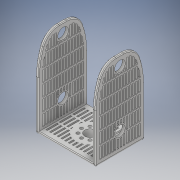
# Autodesk Inventor part: Wheel Case V2
Saved by Autodesk Inventor 2019 (Build 230136000, 136)
## iProperties
Created: 2018-12-01
Part Number: Wheel Case V2
Material: Generic
Document SubType Name: Modeling
Designer: Ashley
Density: 1 g/cm^3
Appearance: Default
Author: Ashley
Autodesk Inventor part; units mm, degrees
ref_plane "YZ Plane" through (0, 0, 0) normal (1, 0, 0) x (0, 1, 0)
ref_plane "XZ Plane" through (0, 0, 0) normal (0, 1, 0) x (-1, 0, 0)
ref_plane "XY Plane" through (0, 0, 0) normal (0, 0, 1) x (1, 0, 0)
sketch "Sketch1" plane through (0, 0, 0) normal (0, 1, 0) x (-1, 0, 0)
  line L0 (40, 32.5) -> (-40, 32.5)
  line L1 (-40, 32.5) -> (-40, -32.5)
  line L2 (-40, -32.5) -> (40, -32.5)
  line L3 (40, -32.5) -> (40, 32.5)
  line L4 (40, 32.5) -> (-40, -32.5) construction
  line L5 (-40, 32.5) -> (40, -32.5) construction
  point P0 (0, 0)
  dimension "d0" = 80
  dimension "d1" = 65
  constraints: 12 end point, 2 midpoint, 2 parallel, 1 horizontal, 1 perpendicular
  measures "d0" distance of L1.end L2.end
  measures "d1" distance of L0.end L1.end
extrude "Top Base Extrusion" add sketch "Sketch1" along normal blind 4
sketch "Sketch2" plane through (0, 4, 0) normal (0, 1, 0) x (1, 0, 0)
  line L0 (-40, -32.5) -> (40, -32.5) construction
  line L1 (40, -32.5) -> (40, 32.5) construction
  line L2 (-40, 32.5) -> (-40, -32.5) construction
  line L3 (-40, 32.5) -> (-36, 32.5)
  line L4 (-36, 32.5) -> (-36, -32.5)
  line L5 (-36, -32.5) -> (-40, -32.5)
  line L6 (-40, -32.5) -> (-40, 32.5)
  line L7 (40, 32.5) -> (36, 32.5)
  line L8 (36, 32.5) -> (36, -32.5)
  line L9 (36, -32.5) -> (40, -32.5)
  line L10 (40, -32.5) -> (40, 32.5)
  point P0 (0, 0)
  dimension "d4" = 4
  dimension "d5" = 4
  constraints: 16 end point, 4 parallel, 2 horizontal, 2 perpendicular, 2 point on line
  measures "d4" distance between parallel lines of L4 L2
  measures "d5" distance between parallel lines of L1 L8
extrude "Side Extrusions" add sketch "Sketch2" along normal blind 110
sketch "Sketch3" plane through (40, 0, 32.5) normal (1, 0, 0) x (0, 0, -1)
  circle A0 centre (32.5, 101.5) radius 7.1
  circle A1 centre (32.5, 26.5) radius 7
  line L0 (65, 0) -> (65, 114) construction
  line L1 (0, 114) -> (65, 114) construction
  line L2 (0, 0) -> (0, 114) construction
  line L3 (0, 4) -> (65, 4) construction
  point P0 (32.5, 0)
  dimension "d8" = 14.2
  dimension "d11" = 101.5
  dimension "d43" = 75
  dimension "d44" = 14
  dimension "d45" = 65
  dimension "d46" = 32.5
  dimension "d47" = 32.5
  dimension "d48" = 32.5
  dimension "d49" = 12.5
  dimension "d50" = 22.5
  constraints: 2 centre point
  measures "d8" diameter of A0
  measures "d11" distance of point (32.5, 0) A0.centre
  measures "d43" distance of A1.centre A0.centre
  measures "d44" diameter of A1
  measures "d45" distance between parallel lines of L2 L0
  measures "d46" distance from line of L0 A0.centre
  measures "d47" distance from line of L2 A0.centre
  measures "d48" distance from line of L0 A1.centre
  measures "d49" distance from line of A0.centre L1
  measures "d50" distance from line of A1.centre L3
extrude "Wheel Axel Hole" cut sketch "Sketch3" against normal up to surface (80 mm away)
sketch "Sketch4" plane through (0, 0, 0) normal (0, -1, 0) x (1, 0, 0)
  circle A0 centre (0, 0) radius 7.1
  circle A1 centre (0, 0) radius 16
  dimension "d16" = 14.2
  dimension "d17" = 32
  constraints: 2 centre point, 2 coincident
  measures "d16" diameter of A0
  measures "d17" diameter of A1
extrude "Chain Interferance Extrusion" add sketch "Sketch4" along normal blind 6
sketch "Sketch5" plane through (0, 0, 0) normal (0, -1, 0) x (1, 0, 0)
  circle A0 centre (0, 0) radius 7.1 construction
  circle A1 centre (0, 0) radius 7.1
  constraints: 1 centre point, 1 coincident, 1 concentric
extrude "Top Center Bearing Hole" cut sketch "Sketch5" against normal up to surface (4 mm away)
sketch "Sketch7" plane through (0, -6, 0) normal (0, -1, 0) x (1, 0, 0)
  circle A0 centre (0, 0) radius 7.1 construction
  circle A1 centre (0, 11.314) radius 2.05
  circle A2 centre (-8.0002, 8.0002) radius 2.05
  circle A3 centre (-11.314, 0) radius 2.05
  circle A4 centre (-8.0002, -8.0002) radius 2.05
  circle A5 centre (0, -11.314) radius 2.05
  circle A6 centre (8.0002, -8.0002) radius 2.05
  circle A7 centre (11.314, 0) radius 2.05
  circle A8 centre (8.0002, 8.0002) radius 2.05
  dimension "d23" = 4.1
  dimension "d24" = 11.314
  dimension "d27" = 360
  constraints: 8 centre point, 17 other
  measures "d23" diameter of A1
  measures "d24" distance of A0.centre A1.centre
extrude "Sprocket Screws Holes" cut sketch "Sketch7" against normal up to next
sketch "Sketch8" plane through (40, 0, 32.5) normal (1, 0, 0) x (0, 0, -1)
  line L0 (65, 0) -> (65, 114) construction
  line L1 (0, 114) -> (65, 114) construction
  line L2 (0, 0) -> (0, 114) construction
  line L3 (65, 91.5) -> (52.0096, 114)
  line L4 (65, 114) -> (0, 114) construction
  line L5 (65, 91.5) -> (90.9808, 91.5) construction
  line L6 (0, 91.5) -> (34.6363, 91.5) construction
  line L7 (0, 91.5) -> (44.4453, 91.5) construction
  line L8 (0, 91.5) -> (12.9904, 114)
  line L9 (65, 91.5) -> (65, 114)
  line L10 (52.0096, 114) -> (65, 114)
  line L11 (12.9904, 114) -> (0, 114)
  line L12 (0, 91.5) -> (0, 114)
  line L13 (0, 91.5) -> (-31.251, 91.5) construction
  point P0 (32.5, 0)
  dimension "d32" = 120
  dimension "d51" = 120
  constraints: 20 end point, 5 point on line, 3 collinear, 3 horizontal, 1 equal length, 1 perpendicular
  measures "d32" angle of L5 L3
  measures "d51" angle of L13 L8
extrude "Side Corners Cut" cut sketch "Sketch8" against normal up to surface (80 mm away)
fillet "Fillet1" radius 95 4 edges at (38, 91.5, 32.5) (-38, 91.5, 32.5) (38, 91.5, -32.5) (-38, 91.5, -32.5)
fillet "Fillet2" radius 23 4 edges at (38, 114, 19.5096) (38, 114, -19.5096) (-38, 114, -19.5096) (-38, 114, 19.5096)
fillet "Fillet3" radius 3 4 edges at (0, 0, -32.5) (-40, 0, 0) (40, 0, 0) (0, 0, 32.5)
fillet "Fillet4" radius 3 1 edges at (-16, 0, 0)
fillet "Fillet5" radius 1 1 edges at (-16, -6, 0)
fillet "Fillet7" radius 1 34 edges at (40, 109.8726, 18.1832) (40, 114, 0) (40, 109.8726, -18.1832) (40, 82.7695, -31.0162) (40, 34.5224, -32.5) (39.1213, 0.8787, -31.6213) (40, 34.5224, 32.5) (39.1213, 0.8787, 31.6213) (40, 82.7695, 31.0162) (36, 35.0224, 32.5) (36, 109.8726, 18.1832) (36, 114, 0) (36, 109.8726, -18.1832) (36, 82.7695, -31.0162) (36, 35.0224, -32.5) (36, 82.7695, 31.0162) (-36, 109.8726, 18.1832) (-36, 114, 0) (-36, 109.8726, -18.1832) (-36, 82.7695, -31.0162) (-36, 35.0224, -32.5) (-36, 35.0224, 32.5) (-36, 82.7695, 31.0162) (-40, 34.5224, 32.5) (-39.1213, 0.8787, 31.6213) (-40, 109.8726, 18.1832) (-40, 114, 0) (-40, 109.8726, -18.1832) (-40, 82.7695, -31.0162) (-40, 34.5224, -32.5) (-39.1213, 0.8787, -31.6213) (-40, 82.7695, 31.0162) (0, 4, 32.5) (0, 4, -32.5)
sketch "Sketch9" plane through (40, 3, -31.5) normal (1, 0, 0) x (0, 0, -1)
  circle A0 centre (-31.5, 98.5) radius 7.1 construction
  circle A1 centre (-31.5, 23.5) radius 7 construction
  line L0 (0, 63.0448) -> (0, 0) construction
  arc A2 (0, 63.0448) -> (-5.8268, 95.6252) centre (-94, 63.0448) ccw construction
  arc A3 (-5.8268, 95.6252) -> (-26.4631, 110) centre (-26.4631, 88) ccw construction
  line L1 (-36.5369, 110) -> (-26.4631, 110) construction
  arc A4 (-36.5369, 110) -> (-57.1732, 95.6252) centre (-36.5369, 88) ccw construction
  arc A5 (-57.1732, 95.6252) -> (-63, 63.0448) centre (31, 63.0448) ccw construction
  line L2 (-63, 0) -> (-63, 63.0448) construction
  line L3 (0, 0) -> (-63, 0) construction
  line L4 (-58.5, 4) -> (-56.5, 4)
  line L5 (-56.5, 4) -> (-56.5, 19)
  line L6 (-56.5, 19) -> (-58.5, 19)
  line L7 (-58.5, 19) -> (-58.5, 4)
  line L8 (-61, -3) -> (-2, -3) construction
  line L9 (-56.5, 36) -> (-58.5, 36)
  line L10 (-58.5, 21) -> (-56.5, 21)
  line L11 (-58.5, 36) -> (-58.5, 21)
  line L12 (-56.5, 21) -> (-56.5, 36)
  line L13 (-56.5, 53) -> (-58.5, 53)
  line L14 (-58.5, 38) -> (-56.5, 38)
  line L15 (-58.5, 53) -> (-58.5, 38)
  line L16 (-56.5, 38) -> (-56.5, 53)
  line L17 (-56.5, 70) -> (-58.5, 70)
  line L18 (-58.5, 55) -> (-56.5, 55)
  line L19 (-58.5, 70) -> (-58.5, 55)
  line L20 (-56.5, 55) -> (-56.5, 70)
  line L21 (-52.5, 19) -> (-54.5, 19)
  line L22 (-54.5, 4) -> (-52.5, 4)
  line L23 (-54.5, 19) -> (-54.5, 4)
  line L24 (-52.5, 4) -> (-52.5, 19)
  line L25 (-52.5, 36) -> (-54.5, 36)
  line L26 (-54.5, 21) -> (-52.5, 21)
  line L27 (-54.5, 36) -> (-54.5, 21)
  line L28 (-52.5, 21) -> (-52.5, 36)
  line L29 (-52.5, 53) -> (-54.5, 53)
  line L30 (-54.5, 38) -> (-52.5, 38)
  line L31 (-54.5, 53) -> (-54.5, 38)
  line L32 (-52.5, 38) -> (-52.5, 53)
  line L33 (-52.5, 70) -> (-54.5, 70)
  line L34 (-54.5, 55) -> (-52.5, 55)
  line L35 (-54.5, 70) -> (-54.5, 55)
  line L36 (-52.5, 55) -> (-52.5, 70)
  line L37 (-48.5, 19) -> (-50.5, 19)
  line L38 (-50.5, 4) -> (-48.5, 4)
  line L39 (-50.5, 19) -> (-50.5, 4)
  line L40 (-48.5, 4) -> (-48.5, 19)
  line L41 (-48.5, 36) -> (-50.5, 36)
  line L42 (-50.5, 21) -> (-48.5, 21)
  line L43 (-50.5, 36) -> (-50.5, 21)
  line L44 (-48.5, 21) -> (-48.5, 36)
  line L45 (-48.5, 53) -> (-50.5, 53)
  line L46 (-50.5, 38) -> (-48.5, 38)
  line L47 (-50.5, 53) -> (-50.5, 38)
  line L48 (-48.5, 38) -> (-48.5, 53)
  line L49 (-48.5, 70) -> (-50.5, 70)
  line L50 (-50.5, 55) -> (-48.5, 55)
  line L51 (-50.5, 70) -> (-50.5, 55)
  line L52 (-48.5, 55) -> (-48.5, 70)
  line L53 (-44.5, 19) -> (-46.5, 19)
  line L54 (-46.5, 4) -> (-44.5, 4)
  line L55 (-46.5, 19) -> (-46.5, 4)
  line L56 (-44.5, 4) -> (-44.5, 19)
  line L57 (-44.5, 36) -> (-46.5, 36)
  line L58 (-46.5, 21) -> (-44.5, 21)
  line L59 (-46.5, 36) -> (-46.5, 21)
  line L60 (-44.5, 21) -> (-44.5, 36)
  line L61 (-44.5, 53) -> (-46.5, 53)
  line L62 (-46.5, 38) -> (-44.5, 38)
  line L63 (-46.5, 53) -> (-46.5, 38)
  line L64 (-44.5, 38) -> (-44.5, 53)
  line L65 (-44.5, 70) -> (-46.5, 70)
  line L66 (-46.5, 55) -> (-44.5, 55)
  line L67 (-46.5, 70) -> (-46.5, 55)
  line L68 (-44.5, 55) -> (-44.5, 70)
  line L69 (-40.5, 19) -> (-42.5, 19)
  line L70 (-42.5, 4) -> (-40.5, 4)
  line L71 (-42.5, 19) -> (-42.5, 4)
  line L72 (-40.5, 4) -> (-40.5, 19)
  line L73 (-40.5, 36) -> (-42.5, 36)
  line L74 (-42.5, 21) -> (-40.5, 21)
  line L75 (-42.5, 36) -> (-42.5, 21)
  line L76 (-40.5, 21) -> (-40.5, 36)
  line L77 (-40.5, 53) -> (-42.5, 53)
  line L78 (-42.5, 38) -> (-40.5, 38)
  line L79 (-42.5, 53) -> (-42.5, 38)
  line L80 (-40.5, 38) -> (-40.5, 53)
  line L81 (-40.5, 70) -> (-42.5, 70)
  line L82 (-42.5, 55) -> (-40.5, 55)
  line L83 (-42.5, 70) -> (-42.5, 55)
  line L84 (-40.5, 55) -> (-40.5, 70)
  line L85 (-52.5, 87) -> (-54.5, 87)
  line L86 (-52.5, 72) -> (-52.5, 87)
  line L87 (-54.5, 87) -> (-54.5, 72)
  line L88 (-54.5, 72) -> (-52.5, 72)
  line L89 (-36.5, 55) -> (-36.5, 70)
  line L90 (-38.5, 70) -> (-38.5, 55)
  line L91 (-38.5, 55) -> (-36.5, 55)
  line L92 (-36.5, 70) -> (-38.5, 70)
  line L93 (-32.5, 55) -> (-32.5, 70)
  line L94 (-34.5, 55) -> (-32.5, 55)
  line L95 (-34.5, 70) -> (-34.5, 55)
  line L96 (-32.5, 70) -> (-34.5, 70)
  line L97 (-28.5, 55) -> (-28.5, 70)
  line L98 (-30.5, 55) -> (-28.5, 55)
  line L99 (-30.5, 70) -> (-30.5, 55)
  line L100 (-28.5, 70) -> (-30.5, 70)
  line L101 (-24.5, 55) -> (-24.5, 70)
  line L102 (-26.5, 55) -> (-24.5, 55)
  line L103 (-26.5, 70) -> (-26.5, 55)
  line L104 (-24.5, 70) -> (-26.5, 70)
  line L105 (-20.5, 55) -> (-20.5, 70)
  line L106 (-22.5, 55) -> (-20.5, 55)
  line L107 (-22.5, 70) -> (-22.5, 55)
  line L108 (-20.5, 70) -> (-22.5, 70)
  line L109 (-16.5, 55) -> (-16.5, 70)
  line L110 (-18.5, 55) -> (-16.5, 55)
  line L111 (-18.5, 70) -> (-18.5, 55)
  line L112 (-16.5, 70) -> (-18.5, 70)
  line L113 (-12.5, 55) -> (-12.5, 70)
  line L114 (-14.5, 55) -> (-12.5, 55)
  line L115 (-14.5, 70) -> (-14.5, 55)
  line L116 (-12.5, 70) -> (-14.5, 70)
  line L117 (-8.5, 55) -> (-8.5, 70)
  line L118 (-10.5, 55) -> (-8.5, 55)
  line L119 (-10.5, 70) -> (-10.5, 55)
  line L120 (-8.5, 70) -> (-10.5, 70)
  line L121 (-4.5, 55) -> (-4.5, 70)
  line L122 (-6.5, 55) -> (-4.5, 55)
  line L123 (-6.5, 70) -> (-6.5, 55)
  line L124 (-4.5, 70) -> (-6.5, 70)
  line L125 (-36.5, 38) -> (-36.5, 53)
  line L126 (-38.5, 38) -> (-36.5, 38)
  line L127 (-38.5, 53) -> (-38.5, 38)
  line L128 (-36.5, 53) -> (-38.5, 53)
  line L129 (-32.5, 38) -> (-32.5, 53)
  line L130 (-34.5, 38) -> (-32.5, 38)
  line L131 (-34.5, 53) -> (-34.5, 38)
  line L132 (-32.5, 53) -> (-34.5, 53)
  line L133 (-28.5, 38) -> (-28.5, 53)
  line L134 (-30.5, 38) -> (-28.5, 38)
  line L135 (-30.5, 53) -> (-30.5, 38)
  line L136 (-28.5, 53) -> (-30.5, 53)
  line L137 (-24.5, 38) -> (-24.5, 53)
  line L138 (-26.5, 38) -> (-24.5, 38)
  line L139 (-26.5, 53) -> (-26.5, 38)
  line L140 (-24.5, 53) -> (-26.5, 53)
  line L141 (-20.5, 38) -> (-20.5, 53)
  line L142 (-22.5, 38) -> (-20.5, 38)
  line L143 (-22.5, 53) -> (-22.5, 38)
  line L144 (-20.5, 53) -> (-22.5, 53)
  line L145 (-16.5, 38) -> (-16.5, 53)
  line L146 (-18.5, 38) -> (-16.5, 38)
  line L147 (-18.5, 53) -> (-18.5, 38)
  line L148 (-16.5, 53) -> (-18.5, 53)
  line L149 (-12.5, 38) -> (-12.5, 53)
  line L150 (-14.5, 38) -> (-12.5, 38)
  line L151 (-14.5, 53) -> (-14.5, 38)
  line L152 (-12.5, 53) -> (-14.5, 53)
  line L153 (-8.5, 38) -> (-8.5, 53)
  line L154 (-10.5, 38) -> (-8.5, 38)
  line L155 (-10.5, 53) -> (-10.5, 38)
  line L156 (-8.5, 53) -> (-10.5, 53)
  line L157 (-4.5, 38) -> (-4.5, 53)
  line L158 (-6.5, 38) -> (-4.5, 38)
  line L159 (-6.5, 53) -> (-6.5, 38)
  line L160 (-4.5, 53) -> (-6.5, 53)
  line L161 (-6.5, 36) -> (-6.5, 21)
  line L162 (-6.5, 21) -> (-4.5, 21)
  line L163 (-4.5, 21) -> (-4.5, 36)
  line L164 (-4.5, 36) -> (-6.5, 36)
  line L165 (-8.5, 21) -> (-8.5, 36)
  line L166 (-10.5, 21) -> (-8.5, 21)
  line L167 (-10.5, 36) -> (-10.5, 21)
  line L168 (-8.5, 36) -> (-10.5, 36)
  line L169 (-12.5, 21) -> (-12.5, 36)
  line L170 (-14.5, 21) -> (-12.5, 21)
  line L171 (-14.5, 36) -> (-14.5, 21)
  line L172 (-12.5, 36) -> (-14.5, 36)
  line L173 (-16.5, 21) -> (-16.5, 36)
  line L174 (-18.5, 21) -> (-16.5, 21)
  line L175 (-18.5, 36) -> (-18.5, 21)
  line L176 (-16.5, 36) -> (-18.5, 36)
  line L177 (-4.5, 4) -> (-4.5, 19)
  line L178 (-6.5, 4) -> (-4.5, 4)
  line L179 (-6.5, 19) -> (-6.5, 4)
  line L180 (-4.5, 19) -> (-6.5, 19)
  line L181 (-8.5, 4) -> (-8.5, 19)
  line L182 (-10.5, 4) -> (-8.5, 4)
  line L183 (-10.5, 19) -> (-10.5, 4)
  line L184 (-8.5, 19) -> (-10.5, 19)
  line L185 (-12.5, 4) -> (-12.5, 19)
  line L186 (-14.5, 4) -> (-12.5, 4)
  line L187 (-14.5, 19) -> (-14.5, 4)
  line L188 (-12.5, 19) -> (-14.5, 19)
  line L189 (-16.5, 4) -> (-16.5, 19)
  line L190 (-18.5, 4) -> (-16.5, 4)
  line L191 (-18.5, 19) -> (-18.5, 4)
  line L192 (-16.5, 19) -> (-18.5, 19)
  line L193 (-22.5, 19) -> (-22.5, 4)
  line L194 (-20.5, 4) -> (-20.5, 19)
  line L195 (-22.5, 4) -> (-20.5, 4)
  line L196 (-20.5, 19) -> (-22.5, 19)
  line L197 (-40.5, 89) -> (-40.5, 104)
  line L198 (-42.5, 104) -> (-42.5, 89)
  line L199 (-42.5, 89) -> (-40.5, 89)
  line L200 (-40.5, 104) -> (-42.5, 104)
  line L201 (-21, 36) -> (-22.9, 36)
  line L202 (-22.9, 36) -> (-22.9, 21)
  line L203 (-22.9, 21) -> (-21, 21)
  line L204 (-21, 21) -> (-21, 36)
  line L205 (-25, 36) -> (-27, 36)
  line L206 (-27, 36) -> (-27, 30.8287)
  line L207 (-25, 29.1312) -> (-25, 36)
  line L208 (-29, 36) -> (-31, 36)
  line L209 (-31, 36) -> (-31, 32.0855)
  line L210 (-29, 31.7286) -> (-29, 36)
  line L211 (-33, 36) -> (-35, 36)
  line L212 (-35, 36) -> (-35, 31.3556)
  line L213 (-33, 31.9682) -> (-33, 36)
  line L214 (-37, 36) -> (-39, 36)
  line L215 (-39, 36) -> (-39, 27.7083)
  line L216 (-39, 4.1699) -> (-37, 4.1699)
  line L217 (-37, 4.1699) -> (-37, 16.8886)
  line L218 (-38.9303, 19.1699) -> (-39, 19.1699)
  line L219 (-39, 19.1699) -> (-39, 4.1699)
  line L220 (-35, 4) -> (-33, 4)
  line L221 (-33, 4) -> (-33, 15.0318)
  line L222 (-35, 15.6444) -> (-35, 4)
  line L223 (-31, 4) -> (-29, 4)
  line L224 (-29, 4) -> (-29, 15.2714)
  line L225 (-31, 14.9145) -> (-31, 4)
  line L226 (-27, 4) -> (-25, 4)
  line L227 (-25, 4) -> (-25, 17.8688)
  line L228 (-27, 16.1713) -> (-27, 4)
  line L229 (-37, 30.1114) -> (-37, 36)
  arc A6 (-25, 29.1312) -> (-27, 30.8287) centre (-31.5, 23.5) ccw
  arc A7 (-29, 31.7286) -> (-31, 32.0855) centre (-31.5, 23.5) ccw
  arc A8 (-33, 31.9682) -> (-35, 31.3556) centre (-31.5, 23.5) ccw
  arc A9 (-37, 30.1114) -> (-39, 27.7083) centre (-31.5, 23.5) ccw
  arc A10 (-38.9303, 19.1699) -> (-37, 16.8886) centre (-31.5, 23.5) ccw
  arc A11 (-35, 15.6444) -> (-33, 15.0318) centre (-31.5, 23.5) ccw
  arc A12 (-31, 14.9145) -> (-29, 15.2714) centre (-31.5, 23.5) ccw
  arc A13 (-27, 16.1713) -> (-25, 17.8688) centre (-31.5, 23.5) ccw
  line L230 (-38.5, 89) -> (-36.5, 89)
  line L231 (-36.5, 89) -> (-36.5, 91.5029)
  line L232 (-38.5, 93.504) -> (-38.5, 89)
  line L233 (-34.5, 89) -> (-32.5, 89)
  line L234 (-32.5, 89) -> (-32.5, 89.9583)
  line L235 (-34.5, 90.4402) -> (-34.5, 89)
  line L236 (-30.5, 89) -> (-28.5, 89)
  line L237 (-28.5, 89) -> (-28.5, 90.4402)
  line L238 (-30.5, 89.9583) -> (-30.5, 89)
  line L239 (-26.5, 89) -> (-24.5, 89)
  line L240 (-24.5, 89) -> (-24.5, 93.504)
  line L241 (-22.5, 89) -> (-20.5, 89)
  line L242 (-20.5, 89) -> (-20.5, 104)
  line L243 (-20.5, 104) -> (-22.5, 104)
  line L244 (-22.5, 104) -> (-22.5, 89)
  line L245 (-14.5, 89) -> (-12.6367, 89)
  line L246 (-12.6367, 89) -> (-12.6367, 99.5253)
  line L247 (-14.5, 101.4494) -> (-14.5, 89)
  line L248 (-18.5, 89) -> (-16.5, 89)
  line L249 (-16.5, 89) -> (-16.5, 102.9913)
  line L250 (-18.5, 104.1428) -> (-18.5, 89)
  line L251 (-26.5, 91.5029) -> (-26.5, 89)
  arc A14 (-30.5, 89.9583) -> (-28.5, 90.4402) centre (-31.5, 98.5) ccw
  arc A15 (-34.5, 90.4402) -> (-32.5, 89.9583) centre (-31.5, 98.5) ccw
  arc A16 (-38.5, 93.504) -> (-36.5, 91.5029) centre (-31.5, 98.5) ccw
  arc A17 (-26.5, 91.5029) -> (-24.5, 93.504) centre (-31.5, 98.5) ccw
  line L252 (-5.8268, 95.6252) -> (-12.7838, 95.6252) construction
  line L253 (1, 63.0448) -> (0, 63.0448) construction
  line L254 (0, 63.0448) -> (-9.3053, 63.0448) construction
  arc A18 (-12.6367, 24.5738) -> (-12.5, 24.8643) centre (-94, 63.0448) ccw
  line L255 (-48.5, 72) -> (-48.5, 87)
  line L256 (-50.5, 87) -> (-50.5, 72)
  line L257 (-48.5, 87) -> (-50.5, 87)
  line L258 (-50.5, 72) -> (-48.5, 72)
  line L259 (-44.5, 72) -> (-44.5, 87)
  line L260 (-46.5, 87) -> (-46.5, 72)
  line L261 (-44.5, 87) -> (-46.5, 87)
  line L262 (-46.5, 72) -> (-44.5, 72)
  line L263 (-40.5, 72) -> (-40.5, 87)
  line L264 (-42.5, 87) -> (-42.5, 72)
  line L265 (-40.5, 87) -> (-42.5, 87)
  line L266 (-42.5, 72) -> (-40.5, 72)
  line L267 (-36.5, 72) -> (-36.5, 87)
  line L268 (-38.5, 87) -> (-38.5, 72)
  line L269 (-36.5, 87) -> (-38.5, 87)
  line L270 (-38.5, 72) -> (-36.5, 72)
  line L271 (-32.5, 72) -> (-32.5, 87)
  line L272 (-34.5, 87) -> (-34.5, 72)
  line L273 (-32.5, 87) -> (-34.5, 87)
  line L274 (-34.5, 72) -> (-32.5, 72)
  line L275 (-28.5, 72) -> (-28.5, 87)
  line L276 (-30.5, 87) -> (-30.5, 72)
  line L277 (-28.5, 87) -> (-30.5, 87)
  line L278 (-30.5, 72) -> (-28.5, 72)
  line L279 (-24.5, 72) -> (-24.5, 87)
  line L280 (-26.5, 87) -> (-26.5, 72)
  line L281 (-24.5, 87) -> (-26.5, 87)
  line L282 (-26.5, 72) -> (-24.5, 72)
  line L283 (-20.5, 72) -> (-20.5, 87)
  line L284 (-22.5, 87) -> (-22.5, 72)
  line L285 (-20.5, 87) -> (-22.5, 87)
  line L286 (-22.5, 72) -> (-20.5, 72)
  line L287 (-16.5, 72) -> (-16.5, 87)
  line L288 (-18.5, 87) -> (-18.5, 72)
  line L289 (-16.5, 87) -> (-18.5, 87)
  line L290 (-18.5, 72) -> (-16.5, 72)
  line L291 (-12.5, 72) -> (-12.5, 87)
  line L292 (-14.5, 87) -> (-14.5, 72)
  line L293 (-12.5, 87) -> (-14.5, 87)
  line L294 (-14.5, 72) -> (-12.5, 72)
  line L295 (-8.5, 72) -> (-8.5, 87)
  line L296 (-10.5, 87) -> (-10.5, 72)
  line L297 (-8.5, 87) -> (-10.5, 87)
  line L298 (-10.5, 72) -> (-8.5, 72)
  line L299 (-6.5, 72) -> (-4.5, 72)
  line L300 (-4.5, 72) -> (-4.5, 72.5185)
  line L301 (-6.5, 84.1102) -> (-6.5, 72)
  line L302 (-10.5, 89) -> (-8.5, 89)
  line L303 (-8.5, 89) -> (-8.5, 91.1473)
  line L304 (-10.5, 96.3175) -> (-10.5, 89)
  arc A19 (-10.1579, 95.6252) -> (-10.5, 96.3175) centre (-26.4631, 88) ccw
  arc A20 (-12.6367, 99.5253) -> (-14.5, 101.4494) centre (-26.4631, 88) ccw
  arc A21 (-16.5, 102.9913) -> (-18.5, 104.1428) centre (-26.4631, 88) ccw
  line L305 (-58.1113, 95.9718) -> (-57.1732, 95.6252) construction
  line L306 (-57.1732, 95.6252) -> (-46.5, 95.6252) construction
  line L307 (-63, 63.0448) -> (-54.1464, 63.0448) construction
  line L308 (-44.5, 89) -> (-46.5, 89)
  line L309 (-46.5, 89) -> (-46.5, 102.9913)
  line L310 (-44.7832, 104) -> (-44.5, 104)
  line L311 (-44.5, 104) -> (-44.5, 89)
  line L312 (-50.5, 89) -> (-48.5, 89)
  line L313 (-48.5, 89) -> (-48.5, 101.4494)
  line L314 (-50.5, 99.3593) -> (-50.5, 89)
  line L315 (-52.5, 89) -> (-54.5, 89)
  line L316 (-54.5, 89) -> (-54.5, 91.1473)
  line L317 (-52.5, 96.3175) -> (-52.5, 89)
  line L318 (-56.5, 72) -> (-58.5, 72)
  line L319 (-58.5, 72) -> (-58.5, 72.5185)
  line L320 (-56.5, 84.1102) -> (-56.5, 72)
  arc A22 (-44.7832, 104) -> (-46.5, 102.9913) centre (-36.5369, 88) ccw
  arc A23 (-48.5, 101.4494) -> (-50.5, 99.3593) centre (-36.5369, 88) ccw
  arc A24 (-52.5, 96.3175) -> (-53.4212, 94.2388) centre (-36.5369, 88) ccw
  arc A25 (-53.4212, 94.2388) -> (-54.5, 91.1473) centre (31, 63.0448) ccw
  arc A26 (-56.5, 84.1102) -> (-58.5, 72.5185) centre (31, 63.0448) ccw
  arc A27 (-4.5, 72.5185) -> (-6.5, 84.1102) centre (-94, 63.0448) ccw
  arc A28 (-8.5, 91.1473) -> (-9.5788, 94.2388) centre (-94, 63.0448) ccw
  arc A29 (-9.5788, 94.2388) -> (-10.5, 96.3175) centre (-26.4631, 88) ccw
  arc A30 (-12.6367, 76.4747) -> (-12.5, 76.6407) centre (-26.4631, 88) ccw
  arc A31 (-12.6367, 99.5253) -> (-14.5, 101.4494) centre (-26.4631, 88) ccw
  arc A32 (-16.5, 102.9913) -> (-18.5, 104.1428) centre (-26.4631, 88) ccw
  point P0 (-31.5, -3)
  point P1 (-40.5, 72)
  point P2 (-40.5, 87)
  point P3 (-42.5, 87)
  point P4 (-42.5, 72)
  point P5 (-54.5, 86.8473)
  point P6 (-50.5, 86.8473)
  point P7 (-46.5, 86.8473)
  point P8 (-42.5, 86.8473)
  point P9 (-38.5, 86.8473)
  point P10 (-34.5, 86.8473)
  point P11 (-30.5, 86.8473)
  point P12 (-26.5, 86.8473)
  point P13 (-22.5, 86.8473)
  point P14 (-18.5, 86.8473)
  point P15 (-14.5, 86.8473)
  point P16 (-10.5, 86.8473)
  dimension "d56" = 2
  dimension "d57" = 15
  dimension "d58" = 4.5
  dimension "d61" = 4
  dimension "d64" = 17
  dimension "d67" = 4
  dimension "d72" = 17
  dimension "d86" = 4
  dimension "d93" = 4
  dimension "d96" = 17
  dimension "d101" = 17
  dimension "d108" = 4
  dimension "d111" = 17
  dimension "d119" = 4
  dimension "d130" = 17
  dimension "d137" = 2
  dimension "d138" = 2
  dimension "d140" = 15
  dimension "d141" = 4.5
  dimension "d147" = 22
  dimension "d152" = 94
  dimension "d157" = 4
  constraints: 628 end point, 54 point on circle, 30 horizontal, 28 parallel, 27 centre point, 26 perpendicular, 22 point on line, 7 coincident, 6 vertical, 479 other
  measures "d56" distance of L5.end L6.end
  measures "d57" distance between parallel lines of L6 L4
  measures "d58" distance between parallel lines of L2 L7
  measures "d61" distance between parallel lines of L3 L4
  measures "d64" distance of L5.end L9.start
  measures "d67" distance of L5.end L21.start
  measures "d72" distance of L33.start L85.start
  measures "d86" distance of L82.end L89.start
  measures "d93" distance of L89.start L93.start
  measures "d96" distance of L89.start L125.start
  measures "d101" distance of L159.start L161.start
  measures "d108" distance of L162.end L165.start
  measures "d111" distance of L162.end L177.start
  measures "d119" distance of L191.start L193.start
  measures "d130" distance of point (-40.5, 72) L197.start
  measures "d137" distance between parallel lines of L206 L210
  measures "d138" distance between parallel lines of L208 L134
  measures "d140" distance of L218.end L216.start
  measures "d141" distance between parallel lines of L0 L177
  measures "d147" radius of A3
  measures "d152" radius of A2
  measures "d157" distance of L86.start L255.start
extrude "Extrusion8" cut sketch "Sketch9" against normal up to surface (80 mm away)
sketch "Sketch10" plane through (0, 0, 0) normal (0, -1, 0) x (1, 0, 0)
  line L0 (-37, 29.5) -> (37, 29.5) construction
  line L1 (-37, -29.5) -> (-37, 29.5) construction
  line L2 (37, -29.5) -> (-37, -29.5) construction
  line L3 (37, 29.5) -> (37, -29.5) construction
  circle A0 centre (0, 0) radius 19 construction
  line L4 (33.5, -25.5) -> (31.5, -25.5)
  line L5 (31.5, -25.5) -> (31.5, -10.5)
  line L6 (31.5, -10.5) -> (33.5, -10.5)
  line L7 (33.5, -10.5) -> (33.5, -25.5)
  line L8 (31.5, -7.5) -> (31.5, 7.5)
  line L9 (33.5, 7.5) -> (33.5, -7.5)
  line L10 (31.5, 7.5) -> (33.5, 7.5)
  line L11 (33.5, -7.5) -> (31.5, -7.5)
  line L12 (31.5, 10.5) -> (31.5, 25.5)
  line L13 (33.5, 25.5) -> (33.5, 10.5)
  line L14 (31.5, 25.5) -> (33.5, 25.5)
  line L15 (33.5, 10.5) -> (31.5, 10.5)
  line L16 (26.5, -25.5) -> (26.5, -10.5)
  line L17 (28.5, -10.5) -> (28.5, -25.5)
  line L18 (26.5, -10.5) -> (28.5, -10.5)
  line L19 (28.5, -25.5) -> (26.5, -25.5)
  line L20 (26.5, -7.5) -> (26.5, 7.5)
  line L21 (28.5, 7.5) -> (28.5, -7.5)
  line L22 (26.5, 7.5) -> (28.5, 7.5)
  line L23 (28.5, -7.5) -> (26.5, -7.5)
  line L24 (26.5, 10.5) -> (26.5, 25.5)
  line L25 (28.5, 25.5) -> (28.5, 10.5)
  line L26 (26.5, 25.5) -> (28.5, 25.5)
  line L27 (28.5, 10.5) -> (26.5, 10.5)
  line L28 (21.5, -25.5) -> (21.5, -10.5)
  line L29 (23.5, -10.5) -> (23.5, -25.5)
  line L30 (21.5, -10.5) -> (23.5, -10.5)
  line L31 (23.5, -25.5) -> (21.5, -25.5)
  line L32 (21.5, -7.5) -> (21.5, 7.5)
  line L33 (23.5, 7.5) -> (23.5, -7.5)
  line L34 (21.5, 7.5) -> (23.5, 7.5)
  line L35 (23.5, -7.5) -> (21.5, -7.5)
  line L36 (21.5, 10.5) -> (21.5, 25.5)
  line L37 (23.5, 25.5) -> (23.5, 10.5)
  line L38 (21.5, 25.5) -> (23.5, 25.5)
  line L39 (23.5, 10.5) -> (21.5, 10.5)
  line L40 (16.5, -25.5) -> (16.5, -10.5)
  line L41 (18.5, -10.5) -> (18.5, -25.5)
  line L42 (16.5, -10.5) -> (18.5, -10.5)
  line L43 (18.5, -25.5) -> (16.5, -25.5)
  line L44 (16.5, 10.5) -> (16.5, 25.5)
  line L45 (16.5, 25.5) -> (18.5, 25.5)
  line L46 (18.5, 10.5) -> (16.5, 10.5)
  line L47 (18.5, 25.5) -> (18.5, 10.5)
  line L48 (13.5, 25.5) -> (11.5, 25.5)
  line L49 (11.5, 25.5) -> (11.5, 15.1245)
  line L50 (13.5, 13.3697) -> (13.5, 25.5)
  line L51 (8.5, 25.5) -> (6.5, 25.5)
  line L52 (6.5, 25.5) -> (6.5, 17.8536)
  line L53 (8.5, 16.9926) -> (8.5, 25.5)
  line L54 (3.5, 25.5) -> (1.5, 25.5)
  line L55 (1.5, 25.5) -> (1.5, 18.9407)
  line L56 (3.5, 18.6748) -> (3.5, 25.5)
  line L57 (-1.5, 25.5) -> (-3.5, 25.5)
  line L58 (-3.5, 25.5) -> (-3.5, 18.6748)
  line L59 (-1.5, 18.9407) -> (-1.5, 25.5)
  line L60 (-6.5, 25.5) -> (-8.5, 25.5)
  line L61 (-8.5, 25.5) -> (-8.5, 16.9926)
  line L62 (-6.5, 17.8536) -> (-6.5, 25.5)
  line L63 (-11.5, 25.5) -> (-13.5, 25.5)
  line L64 (-13.5, 25.5) -> (-13.5, 13.3697)
  line L65 (-11.5, 15.1245) -> (-11.5, 25.5)
  line L66 (-16.5, 25.5) -> (-18.5, 25.5)
  line L67 (-18.5, 25.5) -> (-18.5, 10.5)
  line L68 (-13, 10.5) -> (-11, 10.5)
  line L69 (-16.5, 10.5) -> (-16.5, 25.5)
  line L70 (41.0278, 0) -> (-51.455, 0) construction
  line L71 (-16.5, 10.5) -> (-18.5, 10.5)
  line L72 (-21.5, 25.5) -> (-23.5, 25.5)
  line L73 (-21.5, 10.5) -> (-21.5, 25.5)
  line L74 (-23.5, 25.5) -> (-23.5, 10.5)
  line L75 (-21.5, 10.5) -> (-23.5, 10.5)
  line L76 (-26.5, 25.5) -> (-28.5, 25.5)
  line L77 (-26.5, 10.5) -> (-26.5, 25.5)
  line L78 (-28.5, 25.5) -> (-28.5, 10.5)
  line L79 (-26.5, 10.5) -> (-28.5, 10.5)
  line L80 (-31.5, 25.5) -> (-33.5, 25.5)
  line L81 (-31.5, 10.5) -> (-31.5, 25.5)
  line L82 (-33.5, 25.5) -> (-33.5, 10.5)
  line L83 (-31.5, 10.5) -> (-33.5, 10.5)
  line L84 (-16.5, 0) -> (-16.5, -0.9905)
  line L85 (-18.5, 4.3301) -> (-18.5, 7.5)
  line L86 (-21.5, -7.5) -> (-21.5, 7.5)
  line L87 (-21.5, -7.5) -> (-23.5, -7.5)
  line L88 (-23.5, 7.5) -> (-23.5, -7.5)
  line L89 (-21.5, 7.5) -> (-23.5, 7.5)
  line L90 (-18.5, 7.5) -> (-17.4571, 7.5)
  line L91 (36.0278, 0) -> (-56.455, 0) construction
  line L92 (-28.5, 7.5) -> (-28.5, -7.5)
  line L93 (-26.5, -7.5) -> (-26.5, 7.5)
  line L94 (-26.5, 7.5) -> (-28.5, 7.5)
  line L95 (-26.5, -7.5) -> (-28.5, -7.5)
  line L96 (31.0278, 0) -> (-61.455, 0) construction
  line L97 (-33.5, 7.5) -> (-33.5, -7.5)
  line L98 (-31.5, -7.5) -> (-31.5, 7.5)
  line L99 (-31.5, 7.5) -> (-33.5, 7.5)
  line L100 (-31.5, -7.5) -> (-33.5, -7.5)
  line L101 (41.0278, -18) -> (-51.455, -18) construction
  line L102 (-23.5, -10.5) -> (-23.5, -25.5)
  line L103 (-21.5, -25.5) -> (-21.5, -10.5)
  line L104 (-21.5, -10.5) -> (-23.5, -10.5)
  line L105 (-21.5, -25.5) -> (-23.5, -25.5)
  line L106 (36.0278, -18) -> (-56.455, -18) construction
  line L107 (-28.5, -10.5) -> (-28.5, -25.5)
  line L108 (-26.5, -25.5) -> (-26.5, -10.5)
  line L109 (-26.5, -10.5) -> (-28.5, -10.5)
  line L110 (-26.5, -25.5) -> (-28.5, -25.5)
  line L111 (31.0278, -18) -> (-61.455, -18) construction
  line L112 (-33.5, -10.5) -> (-33.5, -25.5)
  line L113 (-31.5, -25.5) -> (-31.5, -10.5)
  line L114 (-31.5, -10.5) -> (-33.5, -10.5)
  line L115 (-31.5, -25.5) -> (-33.5, -25.5)
  line L116 (-16.5, -25.5) -> (-18.5, -25.5)
  line L117 (-16.5, -25.5) -> (-16.5, -10.5)
  line L118 (-18.5, -10.5) -> (-18.5, -25.5)
  line L119 (-16.5, -10.5) -> (-18.5, -10.5)
  arc A1 (-17.4571, 7.5) -> (-18.5, 4.3301) centre (0, 0) ccw
  line L120 (-18.5, -4.3301) -> (-18.5, -7.5)
  line L121 (-18.5, -7.5) -> (-17.4571, -7.5)
  arc A2 (-18.5, -4.3301) -> (-17.4571, -7.5) centre (0, 0) ccw
  arc A3 (-11.5, 15.1245) -> (-13.5, 13.3697) centre (0, 0) ccw
  arc A4 (-6.5, 17.8536) -> (-8.5, 16.9926) centre (0, 0) ccw
  arc A5 (-1.5, 18.9407) -> (-3.5, 18.6748) centre (0, 0) ccw
  arc A6 (3.5, 18.6748) -> (1.5, 18.9407) centre (0, 0) ccw
  arc A7 (8.5, 16.9926) -> (6.5, 17.8536) centre (0, 0) ccw
  line L122 (18.5, 7.5) -> (17.4571, 7.5)
  line L123 (18.5, 4.3301) -> (18.5, 7.5)
  arc A8 (18.5, 4.3301) -> (17.4571, 7.5) centre (0, 0) ccw
  arc A9 (13.5, 13.3697) -> (11.5, 15.1245) centre (0, 0) ccw
  line L124 (13.5, -25.5) -> (11.5, -25.5)
  line L125 (11.5, -25.5) -> (11.5, -15.1245)
  line L126 (13.5, -13.3697) -> (13.5, -25.5)
  line L127 (8.5, -25.5) -> (6.5, -25.5)
  line L128 (6.5, -25.5) -> (6.5, -17.8536)
  line L129 (8.5, -16.9926) -> (8.5, -25.5)
  line L130 (3.5, -25.5) -> (1.5, -25.5)
  line L131 (1.5, -25.5) -> (1.5, -18.9407)
  line L132 (3.5, -18.6748) -> (3.5, -25.5)
  line L133 (-1.5, -25.5) -> (-3.5, -25.5)
  line L134 (-3.5, -25.5) -> (-3.5, -18.6748)
  line L135 (-1.5, -18.9407) -> (-1.5, -25.5)
  line L136 (-6.5, -25.5) -> (-8.5, -25.5)
  line L137 (-8.5, -25.5) -> (-8.5, -16.9926)
  line L138 (-6.5, -17.8536) -> (-6.5, -25.5)
  line L139 (-11.5, -25.5) -> (-13.5, -25.5)
  line L140 (-13.5, -25.5) -> (-13.5, -13.3697)
  line L141 (-11.5, -15.1245) -> (-11.5, -25.5)
  arc A10 (-13.5, -13.3697) -> (-11.5, -15.1245) centre (0, 0) ccw
  arc A11 (-8.5, -16.9926) -> (-6.5, -17.8536) centre (0, 0) ccw
  arc A12 (-3.5, -18.6748) -> (-1.5, -18.9407) centre (0, 0) ccw
  arc A13 (1.5, -18.9407) -> (3.5, -18.6748) centre (0, 0) ccw
  arc A14 (6.5, -17.8536) -> (8.5, -16.9926) centre (0, 0) ccw
  line L142 (18.5, -7.5) -> (17.4571, -7.5)
  line L143 (18.5, -4.3301) -> (18.5, -7.5)
  arc A15 (17.4571, -7.5) -> (18.5, -4.3301) centre (0, 0) ccw
  arc A16 (11.5, -15.1245) -> (13.5, -13.3697) centre (0, 0) ccw
  point P0 (-19, 0)
  point P1 (19, 0)
  point P2 (-24, 0)
  point P3 (14, 0)
  point P4 (-21.5, 0)
  point P5 (-29, 0)
  point P6 (9, 0)
  point P7 (-26.5, 0)
  point P8 (-19, -18)
  point P9 (19, -18)
  point P10 (-16.5, -18)
  point P11 (-24, -18)
  point P12 (14, -18)
  point P13 (-21.5, -18)
  point P14 (-29, -18)
  point P15 (9, -18)
  point P16 (-26.5, -18)
  dimension "d175" = 2
  dimension "d176" = 15
  dimension "d177" = 4
  dimension "d178" = 3.5
  dimension "d181" = 18
  dimension "d184" = 5
  dimension "d187" = 4
  dimension "d190" = 5
  dimension "d197" = 5
  dimension "d203" = 3
  dimension "d204" = 2
  dimension "d205" = 2
  dimension "d206" = 3
  dimension "d207" = 2
  dimension "d208" = 3
  dimension "d209" = 2
  dimension "d210" = 3
  dimension "d211" = 3
  dimension "d212" = 2
  dimension "d213" = 3
  dimension "d214" = 2
  dimension "d216" = 2
  dimension "d217" = 3
  dimension "d219" = 15
  dimension "d222" = 5
  dimension "d227" = 3.5
  dimension "d230" = 18
  dimension "d235" = 3
  dimension "d237" = 3
  dimension "d239" = 3
  dimension "d242" = 5
  dimension "d245" = 18
  dimension "d250" = 5
  dimension "d255" = 3
  dimension "d256" = 3
  constraints: 280 end point, 32 point on circle, 30 symmetric about line, 18 point on line, 17 horizontal, 16 centre point, 11 parallel, 9 perpendicular, 3 vertical, 1 coincident, 198 other
  measures "d175" distance of L5.end L6.end
  measures "d176" distance of L4.end L5.end
  measures "d177" distance between parallel lines of L4 L2
  measures "d178" distance between parallel lines of L3 L7
  measures "d181" distance of L4.end L8.start
  measures "d184" distance of L4.end L16.start
  measures "d187" distance between parallel lines of L0 L14
  measures "d190" distance of L28.start L40.start
  measures "d197" distance of L36.start L44.start
  measures "d203" distance between parallel lines of L50 L44
  measures "d204" distance of L48.start L48.end
  measures "d205" distance of L51.start L51.end
  measures "d206" distance between parallel lines of L53 L49
  measures "d207" distance of L54.start L54.end
  measures "d208" distance between parallel lines of L56 L52
  measures "d209" distance of L57.start L57.end
  measures "d210" distance between parallel lines of L55 L59
  measures "d211" distance between parallel lines of L58 L62
  measures "d212" distance of L60.start L60.end
  measures "d213" distance between parallel lines of L61 L65
  measures "d214" distance between parallel lines of L64 L65
  measures "d216" distance of L66.start L66.end
  measures "d217" distance between parallel lines of L64 L69
  measures "d219" distance between parallel lines of L66 L71
  measures "d222" distance of L66.start L72.start
  measures "d227" distance between parallel lines of L1 L82
  measures "d230" distance of L72.start L86.end
  measures "d235" distance between parallel lines of L39 L34
  measures "d237" distance between parallel lines of L71 L90
  measures "d239" distance between parallel lines of L86 L85
  measures "d242" distance of L70.start L91.start
  measures "d245" distance of L70.start L101.start
  measures "d250" distance of L103.start L116.start
  measures "d255" distance between parallel lines of L32 L123
  measures "d256" distance between parallel lines of L46 L122
extrude "Extrusion9" cut sketch "Sketch10" against normal up to surface (4 mm away)
body "Solid1" dims "d94" = 20
